Autodesk Inventor part; units mm, degrees
(part 9 of 9)
  arc A551 (-224.1756, -145.2346) -> (-223.6788, -145.732) centre (-223.6434, -145.1998) ccw
  arc A552 (-222.9646, -145.8766) -> (-223.6788, -145.732) centre (-223.8604, -148.4648) ccw
  arc A553 (-222.6756, -148.4414) -> (-222.9646, -145.8766) centre (-223.4324, -147.228) ccw
  arc A554 (-223.3397, -148.7413) -> (-222.6756, -148.4414) centre (-224.1249, -146.1175) ccw
  arc A555 (-223.3397, -148.7413) -> (-223.7134, -149.3368) centre (-223.1868, -149.2523) ccw
  arc A556 (-223.7134, -149.3368) -> (-223.5784, -150.1317) centre (-180.2765, -142.3655) ccw
  arc A557 (-223.5784, -150.1317) -> (-223.0289, -150.5704) centre (-223.0534, -150.0375) ccw
  arc A558 (-222.3031, -150.6341) -> (-223.0289, -150.5704) centre (-222.9035, -153.3063) ccw
  arc A559 (-221.7287, -153.1504) -> (-222.3031, -150.6341) centre (-222.6166, -152.0294) ccw
  arc A560 (-222.3551, -153.5228) -> (-221.7287, -153.1504) centre (-223.4291, -151.0033) ccw
  arc A561 (-222.3551, -153.5228) -> (-222.6598, -154.1564) centre (-222.1459, -154.0134) ccw
  arc A562 (-222.6598, -154.1564) -> (-222.4366, -154.9311) centre (-180.2765, -142.3655) ccw
  arc A563 (-222.4366, -154.9311) -> (-221.8415, -155.3055) centre (-221.9254, -154.7788) ccw
  arc A564 (-221.113, -155.2876) -> (-221.8415, -155.3055) centre (-221.4105, -158.0102) ccw
  arc A565 (-220.2606, -157.7238) -> (-221.113, -155.2876) centre (-221.2683, -156.7092) ccw
  arc A566 (-220.8413, -158.1639) -> (-220.2606, -157.7238) centre (-222.1907, -155.7806) ccw
  arc A567 (-220.8413, -158.1639) -> (-221.0731, -158.8277) centre (-220.5785, -158.6281) ccw
  arc A568 (-221.0731, -158.8277) -> (-220.7646, -159.5726) centre (-180.2765, -142.3655) ccw
  arc A569 (-220.7646, -159.5726) -> (-220.1313, -159.878) centre (-220.2737, -159.3639) ccw
  arc A570 (-219.4094, -159.7786) -> (-220.1313, -159.878) centre (-219.4002, -162.5174) ccw
  arc A571 (-218.2896, -162.104) -> (-219.4094, -159.7786) centre (-219.4046, -161.2086) ccw
  arc A572 (-218.8173, -162.6064) -> (-218.2896, -162.104) centre (-220.4251, -160.3891) ccw
  arc A573 (-218.8173, -162.6064) -> (-218.9734, -163.2919) centre (-218.5042, -163.0382) ccw
  arc A574 (-218.9734, -163.2919) -> (-218.5834, -163.9976) centre (-180.2765, -142.3655) ccw
  arc A575 (-218.5834, -163.9976) -> (-217.9199, -164.2302) centre (-218.119, -163.7353) ccw
  arc A576 (-217.2137, -164.0506) -> (-217.9199, -164.2302) centre (-216.8979, -166.7712) ccw
  arc A577 (-215.8406, -166.236) -> (-217.2137, -164.0506) centre (-217.0488, -165.4711) ccw
  arc A578 (-216.3087, -166.7943) -> (-215.8406, -166.236) centre (-218.1547, -164.771) ccw
  arc A579 (-216.3087, -166.7943) -> (-216.3871, -167.493) centre (-215.9492, -167.1884) ccw
  arc A580 (-216.3871, -167.493) -> (-215.9205, -168.1506) centre (-180.2765, -142.3655) ccw
  arc A581 (-215.9205, -168.1506) -> (-215.2352, -168.3074) centre (-215.4884, -167.8379) ccw
  arc A582 (-214.5535, -168.0499) -> (-215.2352, -168.3074) centre (-213.9351, -170.718) ccw
  arc A583 (-212.9443, -170.0678) -> (-214.5535, -168.0499) centre (-214.2306, -169.443) ccw
  arc A584 (-213.347, -170.6751) -> (-212.9443, -170.0678) centre (-215.4079, -168.8712) ccw
  arc A585 (-213.347, -170.6751) -> (-213.3466, -171.3781) centre (-212.9457, -171.0264) ccw
  arc A586 (-213.3466, -171.3781) -> (-212.8094, -171.9793) centre (-180.2765, -142.3655) ccw
  arc A587 (-212.8094, -171.9793) -> (-212.1108, -172.0584) centre (-212.4149, -171.6203) ccw
  arc A588 (-211.4623, -171.7262) -> (-212.1108, -172.0584) centre (-210.5489, -174.3083) ccw
  arc A589 (-209.6372, -173.5513) -> (-211.4623, -171.7262) centre (-210.9854, -173.0744) ccw
  arc A590 (-209.9694, -174.1998) -> (-209.6372, -173.5513) centre (-212.2193, -172.638) ccw
  arc A591 (-209.9694, -174.1998) -> (-209.8903, -174.8984) centre (-209.5312, -174.504) ccw
  arc A592 (-209.8903, -174.8984) -> (-209.2891, -175.4356) centre (-180.2765, -142.3655) ccw
  arc A593 (-209.2891, -175.4356) -> (-208.5861, -175.436) centre (-208.9374, -175.0347) ccw
  arc A594 (-207.9788, -175.0333) -> (-208.5861, -175.436) centre (-206.7821, -177.4969) ccw
  arc A595 (-205.9609, -176.6425) -> (-207.9788, -175.0333) centre (-207.354, -176.3196) ccw
  arc A596 (-206.2184, -177.3242) -> (-205.9609, -176.6425) centre (-208.629, -176.0241) ccw
  arc A597 (-206.2184, -177.3242) -> (-206.0616, -178.0095) centre (-205.7489, -177.5774) ccw
  arc A598 (-206.0616, -178.0095) -> (-205.404, -178.4761) centre (-180.2765, -142.3655) ccw
  arc A599 (-205.404, -178.4761) -> (-204.7053, -178.3978) centre (-205.0994, -178.0383) ccw
  arc A600 (-204.147, -177.9296) -> (-204.7053, -178.3978) centre (-202.682, -180.2437) ccw
  arc A601 (-201.9616, -179.3027) -> (-204.147, -177.9296) centre (-203.3821, -179.1378) ccw
  arc A602 (-202.1412, -180.0089) -> (-201.9616, -179.3027) centre (-204.6822, -178.9869) ccw
  arc A603 (-202.1412, -180.0089) -> (-201.9086, -180.6724) centre (-201.6463, -180.208) ccw
  arc A604 (-201.9086, -180.6724) -> (-201.2029, -181.0624) centre (-180.2765, -142.3655) ccw
  arc A605 (-201.2029, -181.0624) -> (-200.5174, -180.9064) centre (-200.9492, -180.5932) ccw
  arc A606 (-200.015, -180.3786) -> (-200.5174, -180.9064) centre (-198.3001, -182.5141) ccw
  arc A607 (-197.6896, -181.4984) -> (-200.015, -180.3786) centre (-199.1196, -181.4936) ccw
  arc A608 (-197.789, -182.2203) -> (-197.6896, -181.4984) centre (-200.4284, -181.4892) ccw
  arc A609 (-197.789, -182.2203) -> (-197.4835, -182.8536) centre (-197.2749, -182.3627) ccw
  arc A610 (-197.4835, -182.8536) -> (-196.7387, -183.1621) centre (-180.2765, -142.3655) ccw
  arc A611 (-196.7387, -183.1621) -> (-196.0749, -182.9303) centre (-196.5391, -182.6675) ccw
  arc A612 (-195.6348, -182.3496) -> (-196.0749, -182.9303) centre (-193.6916, -184.2797) ccw
  arc A613 (-193.1986, -183.202) -> (-195.6348, -182.3496) centre (-194.6202, -183.3573) ccw
  arc A614 (-193.2165, -183.9305) -> (-193.1986, -183.202) centre (-195.9212, -183.4995) ccw
  arc A615 (-193.2165, -183.9305) -> (-192.8421, -184.5256) centre (-192.6898, -184.0144) ccw
  arc A616 (-192.8421, -184.5256) -> (-192.0674, -184.7488) centre (-180.2765, -142.3655) ccw
  arc A617 (-192.0674, -184.7488) -> (-191.4338, -184.4441) centre (-191.9244, -184.2349) ccw
  arc A618 (-191.0614, -183.8178) -> (-191.4338, -184.4441) centre (-188.9143, -185.5181) ccw
  arc A619 (-188.5451, -184.3921) -> (-191.0614, -183.8178) centre (-189.9403, -184.7056) ccw
  arc A620 (-188.4814, -185.1179) -> (-188.5451, -184.3921) centre (-191.2173, -184.9925) ccw
  arc A621 (-188.4814, -185.1179) -> (-188.0427, -185.6674) centre (-187.9485, -185.1424) ccw
  arc A622 (-188.0427, -185.6674) -> (-187.2478, -185.8024) centre (-180.2765, -142.3655) ccw
  arc A623 (-187.2478, -185.8024) -> (-186.6523, -185.4287) centre (-187.1633, -185.2758) ccw
  arc A624 (-186.3524, -184.7646) -> (-186.6523, -185.4287) centre (-184.0285, -186.2139) ccw
  arc A625 (-183.7876, -185.0536) -> (-186.3524, -184.7646) centre (-185.139, -185.5214) ccw
  arc A626 (-183.643, -185.7678) -> (-183.7876, -185.0536) centre (-186.3758, -185.9495) ccw
  arc A627 (-183.643, -185.7678) -> (-183.1456, -186.2647) centre (-183.1108, -185.7324) ccw
  arc A628 (-183.1456, -186.2647) -> (-182.3406, -186.3099) centre (-180.2765, -142.3655) ccw
  arc A629 (-182.3406, -186.3099) -> (-181.7907, -185.8718) centre (-182.3156, -185.777) ccw
  arc A630 (-181.567, -185.1783) -> (-181.7907, -185.8718) centre (-179.0954, -186.3583) ccw
  arc A631 (-178.986, -185.1783) -> (-181.567, -185.1783) centre (-180.2765, -185.7944) ccw
  arc A632 (-178.7623, -185.8718) -> (-178.986, -185.1783) centre (-181.4576, -186.3583) ccw
  arc A633 (-178.7623, -185.8718) -> (-178.2124, -186.3099) centre (-178.2374, -185.777) ccw
  arc A634 (-178.2124, -186.3099) -> (-177.4074, -186.2647) centre (-180.2765, -142.3655) ccw
  arc A635 (-177.4074, -186.2647) -> (-176.91, -185.7678) centre (-177.4422, -185.7324) ccw
  arc A636 (-176.7654, -185.0536) -> (-176.91, -185.7678) centre (-174.1772, -185.9495) ccw
  arc A637 (-174.2006, -184.7646) -> (-176.7654, -185.0536) centre (-175.414, -185.5214) ccw
  arc A638 (-173.9007, -185.4287) -> (-174.2006, -184.7646) centre (-176.5245, -186.2139) ccw
  arc A639 (-173.9007, -185.4287) -> (-173.3052, -185.8024) centre (-173.3897, -185.2758) ccw
  arc A640 (-173.3052, -185.8024) -> (-172.5103, -185.6674) centre (-180.2765, -142.3655) ccw
  arc A641 (-172.5103, -185.6674) -> (-172.0716, -185.1179) centre (-172.6045, -185.1424) ccw
  arc A642 (-172.0079, -184.3921) -> (-172.0716, -185.1179) centre (-169.3357, -184.9925) ccw
  arc A643 (-169.4916, -183.8178) -> (-172.0079, -184.3921) centre (-170.6127, -184.7056) ccw
  arc A644 (-169.1192, -184.4441) -> (-169.4916, -183.8178) centre (-171.6387, -185.5181) ccw
  arc A645 (-169.1192, -184.4441) -> (-168.4856, -184.7488) centre (-168.6286, -184.2349) ccw
  arc A646 (-168.4856, -184.7488) -> (-167.7109, -184.5256) centre (-180.2765, -142.3655) ccw
  arc A647 (-167.7109, -184.5256) -> (-167.3365, -183.9305) centre (-167.8632, -184.0144) ccw
  arc A648 (-167.3544, -183.202) -> (-167.3365, -183.9305) centre (-164.6318, -183.4995) ccw
  arc A649 (-164.9183, -182.3496) -> (-167.3544, -183.202) centre (-165.9328, -183.3573) ccw
  arc A650 (-164.4781, -182.9303) -> (-164.9183, -182.3496) centre (-166.8614, -184.2797) ccw
  arc A651 (-164.4781, -182.9303) -> (-163.8143, -183.1621) centre (-164.0139, -182.6675) ccw
  arc A652 (-163.8143, -183.1621) -> (-163.0695, -182.8536) centre (-180.2765, -142.3655) ccw
  arc A653 (-163.0695, -182.8536) -> (-162.764, -182.2203) centre (-163.2781, -182.3627) ccw
  arc A654 (-162.8634, -181.4984) -> (-162.764, -182.2203) centre (-160.1246, -181.4892) ccw
  arc A655 (-160.538, -180.3786) -> (-162.8634, -181.4984) centre (-161.4334, -181.4936) ccw
  arc A656 (-160.0356, -180.9064) -> (-160.538, -180.3786) centre (-162.2529, -182.5141) ccw
  arc A657 (-160.0356, -180.9064) -> (-159.3501, -181.0624) centre (-159.6038, -180.5932) ccw
  arc A658 (-159.3501, -181.0624) -> (-158.6444, -180.6724) centre (-180.2765, -142.3655) ccw
  arc A659 (-158.6444, -180.6724) -> (-158.4118, -180.0089) centre (-158.9067, -180.208) ccw
  arc A660 (-158.5914, -179.3027) -> (-158.4118, -180.0089) centre (-155.8709, -178.9869) ccw
  arc A661 (-156.406, -177.9296) -> (-158.5914, -179.3027) centre (-157.1709, -179.1378) ccw
  arc A662 (-155.8477, -178.3978) -> (-156.406, -177.9296) centre (-157.871, -180.2437) ccw
  arc A663 (-155.8477, -178.3978) -> (-155.149, -178.4761) centre (-155.4536, -178.0383) ccw
  arc A664 (-155.149, -178.4761) -> (-154.4914, -178.0095) centre (-180.2765, -142.3655) ccw
  arc A665 (-154.4914, -178.0095) -> (-154.3346, -177.3242) centre (-154.8041, -177.5774) ccw
  arc A666 (-154.5921, -176.6425) -> (-154.3346, -177.3242) centre (-151.924, -176.0241) ccw
  arc A667 (-152.5742, -175.0333) -> (-154.5921, -176.6425) centre (-153.199, -176.3196) ccw
  arc A668 (-151.967, -175.436) -> (-152.5742, -175.0333) centre (-153.7709, -177.4969) ccw
  arc A669 (-151.967, -175.436) -> (-151.2639, -175.4356) centre (-151.6156, -175.0347) ccw
  arc A670 (-151.2639, -175.4356) -> (-150.6627, -174.8984) centre (-180.2765, -142.3655) ccw
  arc A671 (-150.6627, -174.8984) -> (-150.5836, -174.1998) centre (-151.0218, -174.504) ccw
  arc A672 (-150.9158, -173.5513) -> (-150.5836, -174.1998) centre (-148.3337, -172.638) ccw
  arc A673 (-149.0908, -171.7262) -> (-150.9158, -173.5513) centre (-149.5676, -173.0744) ccw
  arc A674 (-148.4422, -172.0584) -> (-149.0908, -171.7262) centre (-150.0041, -174.3083) ccw
  arc A675 (-148.4422, -172.0584) -> (-147.7436, -171.9793) centre (-148.1381, -171.6203) ccw
  arc A676 (-147.7436, -171.9793) -> (-147.2064, -171.3781) centre (-180.2765, -142.3655) ccw
  arc A677 (-147.2064, -171.3781) -> (-147.206, -170.6751) centre (-147.6073, -171.0264) ccw
  arc A678 (-147.6087, -170.0678) -> (-147.206, -170.6751) centre (-145.1451, -168.8712) ccw
  arc A679 (-145.9995, -168.0499) -> (-147.6087, -170.0678) centre (-146.3224, -169.443) ccw
  arc A680 (-145.3179, -168.3074) -> (-145.9995, -168.0499) centre (-146.618, -170.718) ccw
  arc A681 (-145.3179, -168.3074) -> (-144.6325, -168.1506) centre (-145.0647, -167.8379) ccw
  arc A682 (-144.6325, -168.1506) -> (-144.1659, -167.493) centre (-180.2765, -142.3655) ccw
  arc A683 (-144.1659, -167.493) -> (-144.2443, -166.7943) centre (-144.6038, -167.1884) ccw
  arc A684 (-144.7124, -166.236) -> (-144.2443, -166.7943) centre (-142.3984, -164.771) ccw
  arc A685 (-143.3393, -164.0506) -> (-144.7124, -166.236) centre (-143.5042, -165.4711) ccw
  arc A686 (-142.6331, -164.2302) -> (-143.3393, -164.0506) centre (-143.6551, -166.7712) ccw
  arc A687 (-142.6331, -164.2302) -> (-141.9696, -163.9976) centre (-142.434, -163.7353) ccw
  arc A688 (-141.9696, -163.9976) -> (-141.5796, -163.2919) centre (-180.2765, -142.3655) ccw
  arc A689 (-141.5796, -163.2919) -> (-141.7357, -162.6064) centre (-142.0488, -163.0382) ccw
  arc A690 (-142.2634, -162.104) -> (-141.7357, -162.6064) centre (-140.1279, -160.3891) ccw
  arc A691 (-141.1436, -159.7786) -> (-142.2634, -162.104) centre (-141.1484, -161.2086) ccw
  arc A692 (-140.4217, -159.878) -> (-141.1436, -159.7786) centre (-141.1528, -162.5174) ccw
  arc A693 (-140.4217, -159.878) -> (-139.7884, -159.5726) centre (-140.2793, -159.3639) ccw
  arc A694 (-139.7884, -159.5726) -> (-139.4799, -158.8277) centre (-180.2765, -142.3655) ccw
  arc A695 (-139.4799, -158.8277) -> (-139.7117, -158.1639) centre (-139.9745, -158.6281) ccw
  arc A696 (-140.2924, -157.7238) -> (-139.7117, -158.1639) centre (-138.3623, -155.7806) ccw
  arc A697 (-139.44, -155.2876) -> (-140.2924, -157.7238) centre (-139.2847, -156.7092) ccw
  arc A698 (-138.7115, -155.3055) -> (-139.44, -155.2876) centre (-139.1425, -158.0102) ccw
  arc A699 (-138.7115, -155.3055) -> (-138.1164, -154.9311) centre (-138.6276, -154.7788) ccw
  arc A700 (-138.1164, -154.9311) -> (-137.8932, -154.1564) centre (-180.2765, -142.3655) ccw
  arc A701 (-137.8932, -154.1564) -> (-138.1979, -153.5228) centre (-138.4071, -154.0134) ccw
  arc A702 (-138.8243, -153.1504) -> (-138.1979, -153.5228) centre (-137.1239, -151.0033) ccw
  arc A703 (-138.2499, -150.6341) -> (-138.8243, -153.1504) centre (-137.9364, -152.0294) ccw
  arc A704 (-137.5241, -150.5704) -> (-138.2499, -150.6341) centre (-137.6495, -153.3063) ccw
  arc A705 (-137.5241, -150.5704) -> (-136.9746, -150.1317) centre (-137.4996, -150.0375) ccw
  arc A706 (-136.9746, -150.1317) -> (-136.8396, -149.3368) centre (-180.2765, -142.3655) ccw
  arc A707 (-136.8396, -149.3368) -> (-137.2133, -148.7413) centre (-137.3662, -149.2523) ccw
  arc A708 (-137.8774, -148.4414) -> (-137.2133, -148.7413) centre (-136.4281, -146.1175) ccw
  arc A709 (-137.5884, -145.8766) -> (-137.8774, -148.4414) centre (-137.1207, -147.228) ccw
  arc A710 (-136.8742, -145.732) -> (-137.5884, -145.8766) centre (-136.6926, -148.4648) ccw
  arc A711 (-136.8742, -145.732) -> (-136.3774, -145.2346) centre (-136.9096, -145.1998) ccw
  arc A712 (-136.3774, -145.2346) -> (-136.3322, -144.4296) centre (-180.2765, -142.3655) ccw
  arc A713 (-136.3322, -144.4296) -> (-136.7702, -143.8797) centre (-136.865, -144.4046) ccw
  arc A714 (-137.4637, -143.656) -> (-136.7702, -143.8797) centre (-136.2837, -141.1844) ccw
  arc A715 (-137.4637, -141.075) -> (-137.4637, -143.656) centre (-136.8476, -142.3655) ccw
  arc A716 (-136.7702, -140.8513) -> (-137.4637, -141.075) centre (-136.2837, -143.5466) ccw
  arc A717 (-136.7702, -140.8513) -> (-136.3322, -140.3014) centre (-136.865, -140.3264) ccw
  arc A718 (-136.3322, -140.3014) -> (-136.3774, -139.4964) centre (-180.2765, -142.3655) ccw
  arc A719 (-136.3774, -139.4964) -> (-136.8742, -138.999) centre (-136.9096, -139.5312) ccw
  arc A720 (-137.5884, -138.8544) -> (-136.8742, -138.999) centre (-136.6926, -136.2662) ccw
  arc A721 (-137.8774, -136.2896) -> (-137.5884, -138.8544) centre (-137.1207, -137.503) ccw
  arc A722 (-137.2133, -135.9897) -> (-137.8774, -136.2896) centre (-136.4281, -138.6136) ccw
  arc A723 (-137.2133, -135.9897) -> (-136.8396, -135.3942) centre (-137.3662, -135.4787) ccw
  arc A724 (-136.8396, -135.3942) -> (-136.9746, -134.5993) centre (-180.2765, -142.3655) ccw
  arc A725 (-136.9746, -134.5993) -> (-137.5241, -134.1607) centre (-137.4996, -134.6935) ccw
  arc A726 (-138.2499, -134.0969) -> (-137.5241, -134.1607) centre (-137.6495, -131.4247) ccw
  arc A727 (-138.8243, -131.5806) -> (-138.2499, -134.0969) centre (-137.9364, -132.7017) ccw
  arc A728 (-138.1979, -131.2083) -> (-138.8243, -131.5806) centre (-137.1239, -133.7277) ccw
  arc A729 (-138.1979, -131.2083) -> (-137.8932, -130.5746) centre (-138.4071, -130.7176) ccw
  arc A730 (-137.8932, -130.5746) -> (-138.1164, -129.7999) centre (-180.2765, -142.3655) ccw
  arc A731 (-138.1164, -129.7999) -> (-138.7115, -129.4255) centre (-138.6276, -129.9522) ccw
  arc A732 (-139.44, -129.4434) -> (-138.7115, -129.4255) centre (-139.1425, -126.7208) ccw
  arc A733 (-140.2924, -127.0073) -> (-139.44, -129.4434) centre (-139.2847, -128.0218) ccw
  arc A734 (-139.7117, -126.5671) -> (-140.2924, -127.0073) centre (-138.3623, -128.9504) ccw
  arc A735 (-139.7117, -126.5671) -> (-139.4799, -125.9033) centre (-139.9745, -126.1029) ccw
  arc A736 (-139.4799, -125.9033) -> (-139.7884, -125.1585) centre (-180.2765, -142.3655) ccw
  arc A737 (-139.7884, -125.1585) -> (-140.4217, -124.8531) centre (-140.2793, -125.3671) ccw
  arc A738 (-141.1436, -124.9524) -> (-140.4217, -124.8531) centre (-141.1528, -122.2136) ccw
  arc A739 (-142.2634, -122.627) -> (-141.1436, -124.9524) centre (-141.1484, -123.5224) ccw
  arc A740 (-141.7357, -122.1246) -> (-142.2634, -122.627) centre (-140.1279, -124.3419) ccw
  arc A741 (-141.7357, -122.1246) -> (-141.5796, -121.4391) centre (-142.0488, -121.6928) ccw
  arc A742 (-141.5796, -121.4391) -> (-141.9696, -120.7334) centre (-180.2765, -142.3655) ccw
  arc A743 (-141.9696, -120.7334) -> (-142.6331, -120.5008) centre (-142.434, -120.9957) ccw
  arc A744 (-143.3393, -120.6804) -> (-142.6331, -120.5008) centre (-143.6551, -117.9599) ccw
  arc A745 (-144.7124, -118.495) -> (-143.3393, -120.6804) centre (-143.5042, -119.2599) ccw
  arc A746 (-144.2443, -117.9367) -> (-144.7124, -118.495) centre (-142.3984, -119.96) ccw
  arc A747 (-144.2443, -117.9367) -> (-144.1659, -117.238) centre (-144.6038, -117.5426) ccw
  arc A748 (-144.1659, -117.238) -> (-144.6325, -116.5804) centre (-180.2765, -142.3655) ccw
  arc A749 (-144.6325, -116.5804) -> (-145.3179, -116.4236) centre (-145.0647, -116.8931) ccw
  arc A750 (-145.9995, -116.6811) -> (-145.3179, -116.4236) centre (-146.618, -114.013) ccw
  arc A751 (-147.6087, -114.6632) -> (-145.9995, -116.6811) centre (-146.3224, -115.288) ccw
  arc A752 (-147.206, -114.056) -> (-147.6087, -114.6632) centre (-145.1451, -115.8599) ccw
  arc A753 (-147.206, -114.056) -> (-147.2064, -113.3529) centre (-147.6073, -113.7046) ccw
  arc A754 (-147.2064, -113.3529) -> (-147.7436, -112.7517) centre (-180.2765, -142.3655) ccw
  arc A755 (-147.7436, -112.7517) -> (-148.4422, -112.6726) centre (-148.1381, -113.1108) ccw
  arc A756 (-149.0908, -113.0048) -> (-148.4422, -112.6726) centre (-150.0041, -110.4227) ccw
  arc A757 (-150.9158, -111.1798) -> (-149.0908, -113.0048) centre (-149.5676, -111.6566) ccw
  arc A758 (-150.5836, -110.5312) -> (-150.9158, -111.1798) centre (-148.3337, -112.0931) ccw
  arc A759 (-150.5836, -110.5312) -> (-150.6627, -109.8326) centre (-151.0218, -110.2271) ccw
  arc A760 (-150.6627, -109.8326) -> (-151.2639, -109.2954) centre (-180.2765, -142.3655) ccw
  arc A761 (-151.2639, -109.2954) -> (-151.967, -109.295) centre (-151.6156, -109.6964) ccw
  arc A762 (-152.5742, -109.6977) -> (-151.967, -109.295) centre (-153.7709, -107.2342) ccw
  arc A763 (-154.5921, -108.0885) -> (-152.5742, -109.6977) centre (-153.199, -108.4114) ccw
  arc A764 (-154.3346, -107.4069) -> (-154.5921, -108.0885) centre (-151.924, -108.707) ccw
  arc A765 (-154.3346, -107.4069) -> (-154.4914, -106.7215) centre (-154.8041, -107.1537) ccw
  arc A766 (-154.4914, -106.7215) -> (-155.149, -106.2549) centre (-180.2765, -142.3655) ccw
  arc A767 (-155.149, -106.2549) -> (-155.8477, -106.3333) centre (-155.4536, -106.6928) ccw
  arc A768 (-156.406, -106.8014) -> (-155.8477, -106.3333) centre (-157.871, -104.4874) ccw
  arc A769 (-158.5914, -105.4283) -> (-156.406, -106.8014) centre (-157.1709, -105.5932) ccw
  arc A770 (-158.4118, -104.7221) -> (-158.5914, -105.4283) centre (-155.8709, -105.7441) ccw
  arc A771 (-158.4118, -104.7221) -> (-158.6444, -104.0586) centre (-158.9067, -104.5231) ccw
  arc A772 (-158.6444, -104.0586) -> (-159.3501, -103.6686) centre (-180.2765, -142.3655) ccw
  arc A773 (-159.3501, -103.6686) -> (-160.0356, -103.8247) centre (-159.6038, -104.1378) ccw
  arc A774 (-160.538, -104.3524) -> (-160.0356, -103.8247) centre (-162.2529, -102.2169) ccw
  arc A775 (-162.8634, -103.2326) -> (-160.538, -104.3524) centre (-161.4334, -103.2374) ccw
  arc A776 (-162.764, -102.5107) -> (-162.8634, -103.2326) centre (-160.1246, -103.2418) ccw
  arc A777 (-162.764, -102.5107) -> (-163.0695, -101.8774) centre (-163.2781, -102.3683) ccw
  arc A778 (-163.0695, -101.8774) -> (-163.8143, -101.5689) centre (-180.2765, -142.3655) ccw
  arc A779 (-163.8143, -101.5689) -> (-164.4781, -101.8007) centre (-164.0139, -102.0636) ccw
  arc A780 (-164.9183, -102.3814) -> (-164.4781, -101.8007) centre (-166.8614, -100.4513) ccw
  arc A781 (-167.3544, -101.529) -> (-164.9183, -102.3814) centre (-165.9328, -101.3737) ccw
  arc A782 (-167.3365, -100.8006) -> (-167.3544, -101.529) centre (-164.6318, -101.2315) ccw
  arc A783 (-167.3365, -100.8006) -> (-167.7109, -100.2054) centre (-167.8632, -100.7166) ccw
  arc A784 (-167.7109, -100.2054) -> (-168.4856, -99.9822) centre (-180.2765, -142.3655) ccw
  arc A785 (-168.4856, -99.9822) -> (-169.1192, -100.2869) centre (-168.6286, -100.4961) ccw
  arc A786 (-169.4916, -100.9133) -> (-169.1192, -100.2869) centre (-171.6387, -99.2129) ccw
  arc A787 (-172.0079, -100.3389) -> (-169.4916, -100.9133) centre (-170.6127, -100.0254) ccw
  arc A788 (-172.0716, -99.6131) -> (-172.0079, -100.3389) centre (-169.3357, -99.7385) ccw
  arc A789 (-172.0716, -99.6131) -> (-172.5103, -99.0636) centre (-172.6045, -99.5887) ccw
  arc A790 (-172.5103, -99.0636) -> (-173.3052, -98.9286) centre (-180.2765, -142.3655) ccw
  arc A791 (-173.3052, -98.9286) -> (-173.9007, -99.3023) centre (-173.3897, -99.4552) ccw
  arc A792 (-174.2006, -99.9664) -> (-173.9007, -99.3023) centre (-176.5245, -98.5171) ccw
  arc A793 (-176.7654, -99.6774) -> (-174.2006, -99.9664) centre (-175.414, -99.2097) ccw
  arc A794 (-176.91, -98.9632) -> (-176.7654, -99.6774) centre (-174.1772, -98.7816) ccw
  arc A795 (-176.91, -98.9632) -> (-177.4074, -98.4664) centre (-177.4422, -98.9986) ccw
  arc A796 (-177.4074, -98.4664) -> (-178.2124, -98.4212) centre (-180.2765, -142.3655) ccw
  arc A797 (-178.2124, -98.4212) -> (-178.7623, -98.8592) centre (-178.2374, -98.954) ccw
  arc A798 (-178.986, -99.5527) -> (-178.7623, -98.8592) centre (-181.4576, -98.3727) ccw
  arc A799 (-181.567, -99.5527) -> (-178.986, -99.5527) centre (-180.2765, -98.9366) ccw
  arc A800 (-181.7907, -98.8592) -> (-181.567, -99.5527) centre (-179.0954, -98.3727) ccw
  circle A801 centre (-171.542, -73.2557) radius 25.4
  line L47 (-171.542, -73.2557) -> (-105.9978, 19.434)
  line L48 (-171.542, -73.2557) -> (-150.8033, -87.9208)
  line L49 (-171.542, -73.2557) -> (-192.2807, -58.5906)
  line L50 (-171.6886, -73.4631) -> (-155.4522, -92.9961)
  line L51 (-171.6886, -73.4631) -> (-187.9251, -53.9301)
  line L52 (-171.8353, -73.6705) -> (-161.2076, -96.7402)
  line L53 (-171.8353, -73.6705) -> (-182.463, -50.6008)
  line L54 (-171.6886, -73.4631) -> (-152.1557, -57.2266)
  line L55 (-171.8353, -73.6705) -> (-148.7656, -63.0428)
  line L56 (-171.542, -73.2557) -> (-186.2071, -93.9944)
  line L57 (-171.6886, -73.4631) -> (-191.2216, -89.6995)
  line L58 (-171.8353, -73.6705) -> (-194.905, -84.2982)
  point P0 (-156.8769, -52.517)
  dimension "d906" = 113.5228
  dimension "d907" = 28.5496
  dimension "d908" = 27.94
  dimension "d909" = 42.9717
  dimension "d910" = 44.45
  dimension "d911" = 44.45
  dimension "d912" = 50.8
  dimension "d913" = 28.6487
  dimension "d914" = 0.254
  dimension "d915" = 15
  dimension "d916" = 15
  dimension "d917" = 15
  dimension "d918" = 15
  constraints: 1493 point on circle, 801 centre point, 118 end point, 15 coincident, 9 equal length, 7 midpoint, 5 collinear, 4 tangent, 3 perpendicular, 2 parallel, 1 horizontal, 1 point on line, 6 other
  measures "d906" distance of point (-105.998, 19.434) point (-171.542, -73.256)
  measures "d907" diameter of A457
  measures "d908" distance from line of point (-171.542, -73.256) L32
  measures "d909" diameter of A458
  measures "d910" distance of L43.end L41.start
  measures "d911" distance of L41.start L41.end
  measures "d912" diameter of A801
  measures "d913" diameter of A459
  measures "d914" distance of point (-171.542, -73.256) L50.start
  measures "d915" angle of L48 L50
  measures "d916" angle of L50 L52
  measures "d917" angle of L54 L47
  measures "d918" angle of L55 L54
hole "Hole16" at (0, -73.4631, 171.6886) direction (-1, 0, 0) diameter 29.845 end through all
sketch "Sketch45" plane through (0, 0, 0) normal (1, 0, 0) x (0, 0, -1)
  circle A0 centre (-171.6886, -73.4631) radius 14.9225 projected
  circle A1 centre (-190.7235, -89.2855) radius 2.159 projected
  circle A2 centre (-149.3539, -63.3138) radius 2.159 projected
  circle A3 centre (-161.2076, -96.7402) radius 2.159 projected
  circle A4 centre (-187.9251, -53.9301) radius 2.159 projected
  circle A5 centre (-192.2807, -58.5906) radius 2.159 projected
  circle A6 centre (-157.2508, -53.0458) radius 2.159 projected
  circle A7 centre (-150.8033, -87.9208) radius 2.159 projected
  circle A8 centre (-155.4522, -92.9961) radius 2.159 projected
  circle A9 centre (-182.463, -50.6008) radius 2.159 projected
  circle A10 centre (-152.6538, -57.6407) radius 2.159 projected
  circle A11 centre (-185.8331, -93.4656) radius 2.159 projected
  circle A12 centre (-194.3167, -84.0272) radius 2.159 projected
  arc A13 (-103.9823, -66.1369) -> (-104.5644, -66.2812) centre (-76.4174, -178.6042) ccw projected
  arc A14 (-99.4294, -84.7133) -> (-103.9823, -66.1369) centre (-101.7058, -75.4251) ccw projected
  arc A15 (-99.4294, -84.7133) -> (-99.9153, -84.8337) centre (-76.4174, -178.6042) ccw projected
  arc A16 (-104.5644, -66.2812) -> (-99.9153, -84.8337) centre (-102.2399, -75.5574) ccw projected
  arc A17 (-82.1853, 16.259) -> (-85.3603, 13.084) centre (-82.1853, 13.084) ccw projected
  line L0 (-85.3603, 13.084) -> (-85.3603, 6.734) projected
  arc A18 (-90.1228, 1.9715) -> (-85.3603, 6.734) centre (-90.1228, 6.734) ccw projected
  line L1 (-90.1228, 1.9715) -> (-121.8728, 1.9715) projected
  arc A19 (-126.6353, 6.734) -> (-121.8728, 1.9715) centre (-121.8728, 6.734) ccw projected
  line L2 (-126.6353, 6.734) -> (-126.6353, 13.084) projected
  arc A20 (-126.6353, 13.084) -> (-129.8103, 16.259) centre (-129.8103, 13.084) ccw projected
  line L3 (-129.8103, 16.259) -> (-132.3503, 16.259) projected
  arc A21 (-132.3503, 22.609) -> (-132.3503, 16.259) centre (-132.3503, 19.434) ccw projected
  line L4 (-132.3503, 22.609) -> (-129.8103, 22.609) projected
  arc A22 (-129.8103, 22.609) -> (-126.6353, 25.784) centre (-129.8103, 25.784) ccw projected
  line L5 (-126.6353, 25.784) -> (-126.6353, 32.134) projected
  arc A23 (-121.8728, 36.8965) -> (-126.6353, 32.134) centre (-121.8728, 32.134) ccw projected
  line L6 (-121.8728, 36.8965) -> (-90.1228, 36.8965) projected
  arc A24 (-85.3603, 32.134) -> (-90.1228, 36.8965) centre (-90.1228, 32.134) ccw projected
  line L7 (-85.3603, 32.134) -> (-85.3603, 25.784) projected
  arc A25 (-85.3603, 25.784) -> (-82.1853, 22.609) centre (-82.1853, 25.784) ccw projected
  line L8 (-82.1853, 22.609) -> (-79.6453, 22.609) projected
  arc A26 (-79.6453, 16.259) -> (-79.6453, 22.609) centre (-79.6453, 19.434) ccw projected
  line L9 (-79.6453, 16.259) -> (-82.1853, 16.259) projected
  line L10 (-112.3478, -13.7765) -> (-99.6478, -13.7765) projected
  arc A27 (-99.6478, -18.8819) -> (-99.6478, -13.7765) centre (-99.6478, -16.3292) ccw projected
  line L11 (-99.6478, -18.8819) -> (-112.3478, -18.8819) projected
  arc A28 (-112.3478, -13.7765) -> (-112.3478, -18.8819) centre (-112.3478, -16.3292) ccw projected
  circle A29 centre (-58.8554, 19.434) radius 2.4892 projected
  line L12 (-177.4857, -133.2108) -> (-177.0061, -133.3781) projected
  arc A30 (-183.3071, -151.4366) -> (-177.0061, -133.3781) centre (-180.1566, -142.4074) ccw projected
  line L13 (-183.3071, -151.4366) -> (-183.7867, -151.2692) projected
  arc A31 (-177.4857, -133.2108) -> (-183.7867, -151.2692) centre (-180.6362, -142.24) ccw projected
  circle A32 centre (-76.4174, -178.6042) radius 13.335 projected
  circle A33 centre (-187.1176, -166.8269) radius 2.4892 projected
  circle A34 centre (-174.2102, -166.8866) radius 2.4892 projected
  circle A35 centre (-167.2175, -120.5501) radius 2.4892 projected
  circle A36 centre (-180.1195, -116.9252) radius 2.4892 projected
  circle A37 centre (-193.0957, -120.1058) radius 2.4892 projected
  circle A38 centre (-186.8225, -117.6771) radius 2.4892 projected
  circle A39 centre (-173.4354, -117.9041) radius 2.4892 projected
  circle A40 centre (-168.1768, -164.3742) radius 2.4892 projected
  circle A41 centre (-180.6733, -167.7222) radius 2.4892 projected
  circle A42 centre (-193.0957, -164.2646) radius 2.4892 projected
  circle A43 centre (-85.7798, -94.9817) radius 2.4892 projected
  circle A44 centre (-110.3931, -99.2933) radius 2.4892 projected
  circle A45 centre (-101.8395, -50.0579) radius 2.4892 projected
  circle A46 centre (-124.2369, -62.8574) radius 2.4892 projected
  circle A47 centre (-110.6604, -51.6228) radius 2.4892 projected
  circle A48 centre (-93.2858, -99.3592) radius 2.4892 projected
  circle A49 centre (-118.4334, -56.0666) radius 2.4892 projected
  circle A50 centre (-93.0185, -51.5569) radius 2.4892 projected
  circle A51 centre (-101.8395, -100.8579) radius 2.4892 projected
  circle A52 centre (-80.2428, -88.2574) radius 2.4892 projected
  circle A53 centre (239.2356, -31.496) radius 3.3782 projected
  circle A54 centre (223.7295, 90.3926) radius 3.3782 projected
  circle A55 centre (239.2356, 31.496) radius 3.3782 projected
  circle A56 centre (221.404, -95.9477) radius 3.3782 projected
  line L14 (149.831, -89.2272) -> (89.9434, -38.9755) projected
  arc A57 (88.9, -36.7379) -> (89.9434, -38.9755) centre (91.821, -36.7379) ccw projected
  line L15 (88.9, -36.7379) -> (88.9, -15.621) projected
  arc A58 (91.821, -12.7) -> (88.9, -15.621) centre (91.821, -15.621) ccw projected
  line L16 (91.821, -12.7) -> (174.1799, -12.7) projected
  arc A59 (177.0893, -15.8819) -> (174.1799, -12.7) centre (174.1799, -15.621) ccw projected
  arc A60 (154.2425, -88.4425) -> (177.0893, -15.8819) centre (0, 0) ccw projected
  arc A61 (149.831, -89.2272) -> (154.2425, -88.4425) centre (151.7086, -86.9895) ccw projected
  line L17 (88.9, -0.254) -> (88.9, 0.254) projected
  arc A62 (91.821, 3.175) -> (88.9, 0.254) centre (91.821, 0.254) ccw projected
  line L18 (91.821, 3.175) -> (174.4218, 3.175) projected
  arc A63 (177.3428, 0.254) -> (174.4218, 3.175) centre (174.4218, 0.254) ccw projected
  line L19 (177.3428, 0.254) -> (177.3428, -0.254) projected
  arc A64 (174.4218, -3.175) -> (177.3428, -0.254) centre (174.4218, -0.254) ccw projected
  line L20 (174.4218, -3.175) -> (91.821, -3.175) projected
  arc A65 (88.9, -0.254) -> (91.821, -3.175) centre (91.821, -0.254) ccw projected
  arc A66 (177.0893, 15.8819) -> (169.6939, 53.0738) centre (0, 0) ccw projected
  arc A67 (174.1799, 12.7) -> (177.0893, 15.8819) centre (174.1799, 15.621) ccw projected
  line L21 (174.1799, 12.7) -> (91.821, 12.7) projected
  arc A68 (88.9, 15.621) -> (91.821, 12.7) centre (91.821, 15.621) ccw projected
  line L22 (88.9, 15.621) -> (88.9, 17.1891) projected
  arc A69 (90.5865, 19.8364) -> (88.9, 17.1891) centre (91.821, 17.1891) ccw projected
  line L23 (90.5865, 19.8364) -> (165.6716, 54.8492) projected
  arc A70 (169.6939, 53.0738) -> (165.6716, 54.8492) centre (166.9061, 52.2019) ccw projected
  arc A71 (180.8991, -105.7674) -> (203.0448, 51.8076) centre (0, 0) ccw projected
  arc A72 (204.8485, 54.889) -> (203.0448, 51.8076) centre (205.5059, 52.4355) ccw projected
  line L24 (204.8485, 54.889) -> (206.0753, 55.2177) projected
  arc A73 (209.1938, 53.3924) -> (206.0753, 55.2177) centre (206.7327, 52.7643) ccw projected
  arc A74 (186.3731, -108.9857) -> (209.1938, 53.3924) centre (0, 0) ccw projected
  arc A75 (182.8723, -109.8807) -> (186.3731, -108.9857) centre (184.1805, -107.7035) ccw projected
  line L25 (182.8723, -109.8807) -> (181.7836, -109.2266) projected
  arc A76 (180.8991, -105.7674) -> (181.7836, -109.2266) centre (183.0918, -107.0494) ccw projected
  arc A77 (159.1231, -92.6879) -> (178.5072, 45.237) centre (0, 0) ccw projected
  arc A78 (180.312, 48.3145) -> (178.5072, 45.237) centre (180.9694, 45.861) ccw projected
  line L26 (180.312, 48.3145) -> (181.5388, 48.6432) projected
  arc A79 (184.6584, 46.8139) -> (181.5388, 48.6432) centre (182.1962, 46.1897) ccw projected
  arc A80 (164.6013, -95.8992) -> (184.6584, 46.8139) centre (0, 0) ccw projected
  arc A81 (161.0985, -96.7977) -> (164.6013, -95.8992) centre (162.4067, -94.6205) ccw projected
  line L27 (161.0985, -96.7977) -> (160.0098, -96.1436) projected
  arc A82 (159.1231, -92.6879) -> (160.0098, -96.1436) centre (161.3179, -93.9664) ccw projected
  line L28 (171.9854, -103.3393) -> (170.8967, -102.6851) projected
  arc A83 (170.0112, -99.2275) -> (170.8967, -102.6851) centre (172.2049, -100.5079) ccw projected
  arc A84 (170.0112, -99.2275) -> (190.7761, 48.5222) centre (0, 0) ccw projected
  arc A85 (192.5803, 51.6017) -> (190.7761, 48.5222) centre (193.2377, 49.1483) ccw projected
  line L29 (192.5803, 51.6017) -> (193.8071, 51.9305) projected
  arc A86 (196.9261, 50.1033) -> (193.8071, 51.9305) centre (194.4645, 49.477) ccw projected
  arc A87 (175.4872, -102.4426) -> (196.9261, 50.1033) centre (0, 0) ccw projected
  arc A88 (171.9854, -103.3393) -> (175.4872, -102.4426) centre (173.2936, -101.1621) ccw projected
  circle A89 centre (187.962, 68.4126) radius 2.5527 projected
  circle A90 centre (0, 0) radius 13.335 projected
  circle A91 centre (160.7915, -118.9794) radius 2.5527 projected
  circle A92 centre (145.0649, -113.4346) radius 2.5527 projected
  circle A93 centre (122.2368, -242.899) radius 2.5527 projected
  circle A94 centre (70.3186, -242.899) radius 2.5527 projected
  circle A95 centre (97.9437, -242.899) radius 2.5527 projected
  circle A96 centre (145.0649, -242.899) radius 2.5527 projected
  circle A97 centre (-116.932, -242.899) radius 2.5527 projected
  circle A98 centre (-116.932, -179.399) radius 2.5527 projected
  circle A99 centre (-148.682, -179.399) radius 2.5527 projected
  circle A100 centre (-186.782, -39.699) radius 2.5527 projected
  circle A101 centre (-186.782, -242.899) radius 2.5527 projected
  circle A102 centre (67.218, 63.5) radius 2.5527 projected
  circle A103 centre (-59.782, 63.5) radius 2.5527 projected
  circle A104 centre (-8.982, 63.5) radius 2.5527 projected
  circle A105 centre (143.418, 63.5) radius 2.5527 projected
  circle A106 centre (-186.782, -179.399) radius 2.5527 projected
  circle A107 centre (-148.682, -39.699) radius 2.5527 projected
  circle A108 centre (-116.932, -39.699) radius 2.5527 projected
  circle A109 centre (-148.682, -242.899) radius 2.5527 projected
  circle A110 centre (11.1125, -19.2474) radius 2.2479 projected
  circle A111 centre (-22.225, 0) radius 2.2479 projected
  circle A112 centre (11.1125, 19.2474) radius 2.2479 projected
  circle A113 centre (22.225, 0) radius 2.2479 projected
  circle A114 centre (-11.1125, 19.2474) radius 2.2479 projected
  circle A115 centre (-11.1125, -19.2474) radius 2.2479 projected
  line L30 (-80.5978, 54.7781) -> (-131.3978, 54.7781) projected
  arc A116 (-131.3978, 59.8835) -> (-131.3978, 54.7781) centre (-131.3978, 57.3308) ccw projected
  line L31 (-131.3978, 59.8835) -> (-80.5978, 59.8835) projected
  arc A117 (-80.5978, 54.7781) -> (-80.5978, 59.8835) centre (-80.5978, 57.3308) ccw projected
  circle A118 centre (-123.52, 44.45) radius 2.4892 projected
  arc A119 (-166.8187, -7.1514) -> (-170.0188, -10.965) centre (-168.4187, -9.0582) ccw projected
  arc A120 (-166.8187, -7.1514) -> (-135.2171, -21.8874) centre (-123.52, 44.45) ccw projected
  arc A121 (-136.0816, -26.7902) -> (-135.2171, -21.8874) centre (-135.6494, -24.3388) ccw projected
  arc A122 (-170.0188, -10.965) -> (-136.0816, -26.7902) centre (-123.52, 44.45) ccw projected
  arc A123 (-196.307, 76.2) -> (-199.482, 73.025) centre (-196.307, 73.025) ccw projected
  line L32 (-199.482, 73.025) -> (-199.482, -252.424) projected
  arc A124 (-199.482, -252.424) -> (-196.307, -255.599) centre (-196.307, -252.424) ccw projected
  line L33 (-196.307, -255.599) -> (147.8383, -255.599) projected
  arc A125 (147.8383, -255.599) -> (150.6952, -253.8092) centre (147.8383, -252.424) ccw projected
  line L34 (194.4526, -163.563) -> (150.6952, -253.8092) projected
  arc A126 (194.8736, -162.9119) -> (194.4526, -163.563) centre (197.3095, -164.9483) ccw projected
  arc A127 (194.8736, -162.9119) -> (235.5329, 95.0804) centre (0, 0) ccw projected
  arc A128 (235.5329, 95.0804) -> (218.389, 101.8364) centre (223.7562, 90.3263) ccw projected
  line L35 (218.389, 101.8364) -> (173.6183, 80.9596) projected
  arc A129 (152.1493, 76.2) -> (173.6183, 80.9596) centre (152.1493, 127) ccw projected
  line L36 (152.1493, 76.2) -> (-196.307, 76.2) projected
  circle A130 centre (-150.8033, -87.9208) radius 2.159 projected
  circle A131 centre (-161.2076, -96.7402) radius 2.159 projected
  constraints: 6 coincident
hole "Hole17" at (0, -87.9208, 150.8033) at (0, -92.9961, 155.4522) at (0, -96.7402, 161.2076) at (0, -58.5906, 192.2807) at (0, -53.9301, 187.9251) at (0, -50.6008, 182.463) direction (-1, 0, 0) diameter 4.9784 end through all clearance for "Flat Head Machine Screw (82)" size "#10" standard "Ansi Unified Screw Threads"
sketch "Sketch46" plane through (-3.175, 0, 0) normal (-1, 0, 0) x (0, 0, 1)
  circle A0 centre (-68.4657, -246.5874) radius 67.7037
  line L0 (259.6346, -316.0887) -> (-46.0359, -182.4022)
  line L1 (-147.8383, -255.599) -> (196.307, -255.599) projected
  line L2 (-194.4526, -163.563) -> (-150.6952, -253.8092) projected
  arc A1 (-150.6952, -253.8092) -> (-147.8383, -255.599) centre (-147.8383, -252.424) ccw projected
  line L3 (137.1736, -255.599) -> (-43.1816, -176.7197)
  arc A2 (-43.1816, -176.7197) -> (-144.6657, -255.599) centre (-72.4908, -243.7343) ccw
  line L4 (-144.6657, -255.599) -> (137.1736, -255.599)
  point P0 (0, 0)
  dimension "d935" = 6.35
  dimension "d936" = 196.85
  dimension "d937" = 76.2
  constraints: 6 end point, 2 centre point, 2 point on circle, 2 point on line, 1 collinear, 1 parallel, 1 tangent, 5 other
  measures "d935" distance between parallel lines of L0 L3
  measures "d936" distance of L3.start L3.end
  measures "d937" horizontal distance of L4.start A0.centre
extrude "Extrusion25" cut sketch "Sketch46" against normal blind 3.175 contours A0 L1 | A0 L1 A2 L3 picked at (-70.05, -225.393)
sketch "Sketch47" plane through (-3.175, 0, 0) normal (-1, 0, 0) x (0, 0, 1)
  circle A0 centre (-145.0649, -194.74) radius 2.5527
  circle A1 centre (-145.0649, -113.4346) radius 2.5527 projected
  point P0 (0, 0)
  dimension "d940" = 5.1054
  dimension "d941" = 76.2
  dimension "d942" = 0
  constraints: 1 centre point
  measures "d940" diameter of A0
  measures "d942" horizontal distance of A1.centre A0.centre
extrude "Extrusion26" cut sketch "Sketch47" against normal blind 3.175 contours A0
equation "\"d21\" = d20"
equation "\"d22\" = d20"
equation "\"d23\" = d20"
equation "\"d34\" = d33"
equation "\"d82\" = 0.5 * d81"
equation "\"d83\" = d72"
equation "\"d88\" = d72"
equation "\"d90\" = d74"
equation "\"d91\" = d76"
equation "\"d95\" = 0.5 * d94"
equation "\"d103\" = 0.5 * d100"
equation "\"d104\" = d35"
equation "\"d130\" = d35"
equation "\"d193\" = d192"
equation "\"d35\" = 3.175"
body "Solid1"
